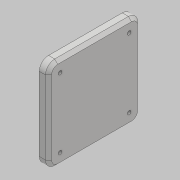
# Autodesk Inventor part: exercise2-5
Saved by Autodesk Inventor 2018 (Build 220112000, 112)
## iProperties
Created: 2020-09-21
Part Number: exercise2-5
Material: 一般
Document SubType Name: Modeling
Designer: 王鼎鈞
Density: 1 g/cm^3
Appearance: 預設
Author: 王鼎鈞
Autodesk Inventor part; units mm, degrees
ref_plane "YZ Plane" through (0, 0, 0) normal (1, 0, 0) x (0, 1, 0)
ref_plane "XZ Plane" through (0, 0, 0) normal (0, 1, 0) x (-1, 0, 0)
ref_plane "XY Plane" through (0, 0, 0) normal (0, 0, 1) x (1, 0, 0)
sketch "草圖1" plane through (0, 0, 0) normal (1, 0, 0) x (0, 1, 0)
  line L0 (-210, 0) -> (210, 0) projected
  line L1 (0, -210) -> (0, 210) projected
  line L2 (-150, 150) -> (150, 150)
  line L3 (150, 150) -> (150, -150)
  line L4 (150, -150) -> (-150, -150)
  line L5 (-150, -150) -> (-150, 150)
  line L6 (-150, 150) -> (150, -150) construction
  line L7 (150, 150) -> (-150, -150) construction
  point P0 (0, 0)
  dimension "d0" = 300
  dimension "d1" = 300
  constraints: 12 end point, 2 midpoint, 2 parallel, 1 horizontal, 1 perpendicular
  measures "d0" distance of L3.end L4.end
  measures "d1" distance of L2.end L3.end
extrude "擠出1" add sketch "草圖1" along normal blind 30
fillet "圓角1" radius 30 4 edges at (15, -150, 150) (15, -150, -150) (15, 150, 150) (15, 150, -150)
chamfer "倒角1" distance 10 angle 45 8 edges at (30, -150, 0) (30, -141.2132, -141.2132) (30, 0, -150) (30, 141.2132, -141.2132) (30, 150, 0) (30, 141.2132, 141.2132) (30, 0, 150) (30, -141.2132, 141.2132)
sketch "草圖2" plane through (30, 0, 0) normal (1, 0, 0) x (0, 0, -1)
  line L0 (0, -210) -> (0, 210) projected
  line L1 (210, 0) -> (-210, 0) projected
  line L2 (-112.5, -210) -> (-112.5, 210)
  line L3 (210, 112.5) -> (-210, 112.5)
  line L4 (-112.5, -112.5) -> (112.5, -112.5)
  line L5 (112.5, -112.5) -> (112.5, 112.5)
  line L6 (112.5, 112.5) -> (-112.5, 112.5)
  line L7 (-112.5, 112.5) -> (-112.5, -112.5)
  line L8 (-112.5, -112.5) -> (112.5, 112.5) construction
  line L9 (112.5, -112.5) -> (-112.5, 112.5) construction
  point P0 (0, 0)
  dimension "d8" = 112.5
  dimension "d9" = 112.5
  dimension "d17" = 225
  dimension "d18" = 225
  constraints: 16 end point, 4 parallel, 3 coincident, 2 midpoint, 2 point on line, 1 horizontal, 1 perpendicular
  measures "d8" distance between parallel lines of L0 L2
  measures "d9" distance between parallel lines of L1 L3
  measures "d17" distance of L6.end L5.end
  measures "d18" distance of L5.end L4.end
hole "孔1" at (30, 112.5, 112.5) direction (-1, 0, 0) diameter 12 depth 10 tip angle 118
hole "孔2" at (30, 112.5, -112.5) at (30, -112.5, -112.5) at (30, -112.5, 112.5) direction (-1, 0, 0) diameter 12 depth 10 tip angle 118
sketch "草圖3" plane through (0, 0, 0) normal (-1, 0, 0) x (0, 0, 1)
  arc A0 (-120, 150) -> (-150, 120) centre (-120, 120) ccw projected
  line L0 (-150, 120) -> (-150, -120) projected
  arc A1 (-150, -120) -> (-120, -150) centre (-120, -120) ccw projected
  line L1 (-120, -150) -> (120, -150) projected
  arc A2 (120, -150) -> (150, -120) centre (120, -120) ccw projected
  line L2 (150, -120) -> (150, 120) projected
  arc A3 (150, 120) -> (120, 150) centre (120, 120) ccw projected
  line L3 (120, 150) -> (-120, 150) projected
  line L4 (120, -120) -> (-120, -120)
  line L5 (-120, -120) -> (-120, 120)
  line L6 (-120, 120) -> (120, 120)
  line L7 (120, 120) -> (120, -120)
  point P0 (0, 0)
  dimension "d26" = 30
  constraints: 8 end point, 4 coincident, 3 other
  measures "d26" distance between parallel lines of L1 L4
hole "孔3" at (0, -120, 120) at (0, 120, 120) at (0, 120, -120) at (0, -120, -120) direction (1, 0, 0) diameter 12 depth 10 tip angle 118
